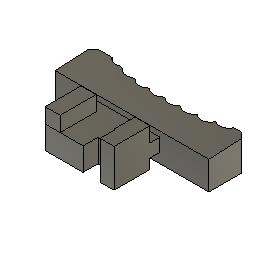
pwrtech_button (Autodesk Fusion 360 design; units mm, degrees)
Autodesk Fusion 360 part; units mm, degrees
note: some values were not read from the file. Chosen so that the rebuilt part matches the saved one: a direction; which face or edge a step refers to; the sign of a taper.
sketch "Sketch1" plane through (0, 0, 0) normal (0, 0, 1) x (1, 0, 0)
  line L0 (0, 0) -> (15.4, 0)
  line L1 (15.4, 0) -> (15.4, -1.3)
  line L2 (0, 0) -> (0, -1.3)
  line L3 (15.4, -1.3) -> (10.5, -1.3)
  line L4 (10.5, -1.3) -> (10.5, -5.9)
  line L5 (0, -1.3) -> (3.6, -1.3)
  line L6 (10.5, -5.9) -> (9, -5.9)
  line L7 (9, -5.9) -> (9, -4.4)
  line L8 (9, -4.4) -> (7.5, -4.4)
  line L9 (7.5, -4.4) -> (7.5, -5.9)
  line L10 (3.6, -1.3) -> (3.6, -5.9)
  line L11 (7.5, -5.9) -> (3.6, -5.9)
  line L12 (10.5, -1.3) -> (10.5, -2.3)
  line L13 (10.5, -2.3) -> (9, -2.3)
  line L14 (9, -2.3) -> (9, -4.4)
  line L15 (9, -4.4) -> (10.5, -4.4)
  line L16 (10.5, -4.4) -> (10.5, -2.3)
  line L17 (3.6, -2.3) -> (5.1, -2.3)
  line L18 (5.1, -2.3) -> (5.1, -4.4)
  line L19 (5.1, -4.4) -> (3.6, -4.4)
  line L20 (3.6, -4.4) -> (3.6, -2.3)
  line L21 (3.6, -1.3) -> (3.6, -3.1)
  line L22 (3.6, -3.1) -> (5.1, -3.1)
  line L23 (5.1, -3.1) -> (5.1, -5.2)
  line L24 (5.1, -5.2) -> (3.6, -5.2)
  line L25 (3.6, -5.2) -> (3.6, -3.1)
  line L26 (10.5, -1.3) -> (10.5, -3.1)
  line L27 (10.5, -3.1) -> (9, -3.1)
  line L28 (9, -3.1) -> (9, -5.2)
  line L29 (9, -5.2) -> (10.5, -5.2)
  line L30 (10.5, -5.2) -> (10.5, -3.1)
  dimension "d1" = 15.4
  dimension "d2" = 1.3
  dimension "d3" = 1.3
  dimension "d4" = 4.9
  dimension "d5" = 4.6
  dimension "d6" = 3.6
  dimension "d7" = 1.5
  dimension "d8" = 1.5
  dimension "d9" = 1.5
  dimension "d10" = 1.5
  dimension "d11" = 1
  dimension "d12" = 1.5
  dimension "d13" = 2.1
  dimension "d14" = 1.8
  dimension "d15" = 1.5
  dimension "d16" = 2.1
  dimension "d17" = 1.8
  dimension "d18" = 1.5
  dimension "d19" = 2.1
  constraint coincident L0.start L2.start
  constraint horizontal L0
  constraint perpendicular L0 L1
  constraint perpendicular L0 L2
  constraint perpendicular L1 L3
  constraint perpendicular L3 L4
  constraint perpendicular L2 L5
  constraint perpendicular L4 L6
  constraint perpendicular L6 L7
  constraint perpendicular L7 L8
  constraint perpendicular L8 L9
  constraint perpendicular L5 L10
  constraint perpendicular L3 L12
  constraint horizontal L13
  constraint vertical L14
  constraint horizontal L15
  constraint vertical L16
  constraint horizontal L17
  constraint vertical L18
  constraint horizontal L19
  constraint vertical L20
  constraint coincident L10 L17.start
  constraint perpendicular L17 L21
  constraint horizontal L22
  constraint vertical L23
  constraint horizontal L24
  constraint vertical L25
  constraint vertical L26
  constraint horizontal L27
  constraint vertical L28
  constraint horizontal L29
  constraint vertical L30
  measures "d1" distance of L0.start L0.end
  measures "d2" distance of L0.end L1.end
  measures "d3" distance of L0.start L2.end
  measures "d4" distance of L1.end L3.end
  measures "d5" distance of L3.end L4.end
  measures "d6" distance of L2.end L5.end
  measures "d7" distance of L4.end L6.end
  measures "d8" distance of L6.end L7.end
  measures "d9" distance of L7.end L8.end
  measures "d10" distance of L8.end L9.end
  measures "d11" distance of L3.end L12.end
  measures "d12" distance of L17.start L17.end
  measures "d13" distance of L17.start L19.end
  measures "d14" distance of L5.end L21.end
  measures "d15" distance of L21.end L22.end
  measures "d16" distance of L21.end L24.end
  measures "d17" distance of L3.end L26.end
  measures "d18" distance of L26.end L27.end
  measures "d19" distance of L26.end L29.end
extrude "Extrude1" add sketch "Sketch1" along normal blind 2 makes body 1
extrude "Extrude2" add sketch "Sketch1" along normal blind 3 contours L10 L17 L18 L20 L21 L22 | L4 L13 L14 L16 L26 L27 | L10 L18 L19 L20 L22 L23 L25 | L4 L14 L15 L16 L27 L28 L30 bodies 1
extrude "Extrude3" cut sketch "Sketch1" along normal blind 0.5 contours L10 L17 L18 L20 L21 L22 | L4 L13 L14 L16 L26 L27 bodies 1
extrude "Extrude4" cut 2 faces at (4.1, -2.3, 0.1667) (10, -2.3, 0.1667) along direction (0, 1, 0) blind 1 on bodies 1 bodies 1
extrude "Extrude5" cut 1 faces at (5.1, -1.9, 0.1667) along direction (1, 0, 0) blind 6.5 on bodies 1 bodies 1
extrude "Extrude6" cut 1 faces at (9, -4.9, 1.3333) along direction (1, 0, 0) blind 0.1 on bodies 1 bodies 1
extrude "Extrude7" cut 1 faces at (7.5, -5.4, 1.3333) along direction (-1, 0, 0) blind 0.1 on bodies 1 bodies 1
extrude "Extrude8" add 1 faces at (5.1333, 0, 0.6667) along direction (0, 1, 0) blind 2.5 on bodies 1 bodies 1
sketch "Sketch2" plane through (0, 0, 2) normal (0, 0, 1) x (-1, 0, 0)
  line L0 (-7.4, 4.4) -> (-9, 4.4)
  line L1 (-9, 4.4) -> (-9, 2.3)
  line L2 (-9, 2.3) -> (-10.5, 2.3)
  line L3 (-10.5, 2.3) -> (-10.5, 1.3)
  line L4 (-10.5, 1.3) -> (-15.4, 1.3)
  line L5 (-15.4, 1.3) -> (-15.4, -2.5)
  line L6 (-15.4, -2.5) -> (0, -2.5)
  line L7 (0, -2.5) -> (0, 1.3)
  line L8 (0, 1.3) -> (-3.6, 1.3)
  line L9 (-3.6, 1.3) -> (-3.6, 2.3)
  line L10 (-3.6, 2.3) -> (-5.1, 2.3)
  line L11 (-5.1, 2.3) -> (-5.1, 4.4)
  line L12 (-5.1, 4.4) -> (-3.6, 4.4)
  line L13 (-3.6, 4.4) -> (-3.6, 5.9)
  line L14 (-3.6, 5.9) -> (-7.4, 5.9)
  line L15 (-7.4, 5.9) -> (-7.4, 4.4)
  spline S0 degree 5 poles (-13.1932, -2.5) (-13.16, -2.4751) (-13.0906, -2.4264) (-12.9777, -2.3563) (-12.8094, -2.2687) (-12.5691, -2.1693) (-12.2987, -2.0801) (-11.9976, -2.0011) (-11.6653, -1.9325) (-11.3014, -1.8744) (-10.9061, -1.8266) (-10.4808, -1.7887) (-10.0277, -1.7597) (-9.551, -1.7384) (-9.0559, -1.723) (-8.5481, -1.712) (-8.0339, -1.7042) (-7.5194, -1.6992) (-7.0101, -1.6972) (-6.5106, -1.6999) (-6.0246, -1.7099) (-5.5551, -1.7299) (-5.1045, -1.7625) (-4.6748, -1.8092) (-4.2679, -1.8704) (-3.8854, -1.9443) (-3.5289, -2.0272) (-3.1998, -2.1149) (-2.8992, -2.2029) (-2.6279, -2.2874) (-2.3864, -2.366) (-2.217, -2.4233) (-2.1033, -2.4629) (-2.0335, -2.4879) (-2, -2.5) knots 0 0 0 0 0 0 0.033333 0.066667 0.1 0.133333 0.166667 0.2 0.233333 0.266667 0.3 0.333333 0.366667 0.4 0.433333 0.466667 0.5 0.533333 0.566667 0.6 0.633333 0.666667 0.7 0.733333 0.766667 0.8 0.833333 0.866667 0.9 0.933333 0.966667 1 1 1 1 1 1
  point P0 (-10.5113, -1.7938)
  point P1 (-4.5685, -1.8279)
  point P2 (-7.415, -1.6993)
  point P3 (-12.319, -2.091)
  point P4 (-2.8487, -2.2195)
  constraint coincident L6 S0.start
  constraint coincident L6 S0.end
extrude "Extrude9" cut sketch "Sketch2" against normal blind 2 contours L6 S0 bodies 1
chamfer "Chamfer1" distance 0.5 angle 45 2 edges at (0, 2.5, 1) (15.4, 2.5, 1) on bodies 1
sketch "Sketch3" plane through (0, 0, 2) normal (0, 0, 1) x (-1, 0, 0)
  line L0 (-15.4, -2) -> (-14.9, -2.5)
  line L1 (-14.9, -2.5) -> (-13.1932, -2.5)
  spline S0 degree 5 poles (-13.1932, -2.5) (-13.16, -2.4751) (-13.0906, -2.4264) (-12.9777, -2.3563) (-12.8094, -2.2687) (-12.5691, -2.1693) (-12.2987, -2.0801) (-11.9976, -2.0011) (-11.6653, -1.9325) (-11.3014, -1.8744) (-10.9061, -1.8266) (-10.4808, -1.7887) (-10.0277, -1.7597) (-9.551, -1.7384) (-9.0559, -1.723) (-8.5481, -1.712) (-8.0339, -1.7042) (-7.5194, -1.6992) (-7.0101, -1.6972) (-6.5106, -1.6999) (-6.0246, -1.7099) (-5.5551, -1.7299) (-5.1045, -1.7625) (-4.6748, -1.8092) (-4.2679, -1.8704) (-3.8854, -1.9443) (-3.5289, -2.0272) (-3.1998, -2.1149) (-2.8992, -2.2029) (-2.6279, -2.2874) (-2.3864, -2.366) (-2.217, -2.4233) (-2.1033, -2.4629) (-2.0335, -2.4879) (-2, -2.5) knots 0 0 0 0 0 0 0.033333 0.066667 0.1 0.133333 0.166667 0.2 0.233333 0.266667 0.3 0.333333 0.366667 0.4 0.433333 0.466667 0.5 0.533333 0.566667 0.6 0.633333 0.666667 0.7 0.733333 0.766667 0.8 0.833333 0.866667 0.9 0.933333 0.966667 1 1 1 1 1 1
  line L2 (-2, -2.5) -> (-0.5, -2.5)
  line L3 (-0.5, -2.5) -> (0, -2)
  line L4 (0, -2) -> (0, 1.3)
  line L5 (0, 1.3) -> (-3.6, 1.3)
  line L6 (-3.6, 1.3) -> (-3.6, 2.3)
  line L7 (-3.6, 2.3) -> (-5.1, 2.3)
  line L8 (-5.1, 2.3) -> (-5.1, 4.4)
  line L9 (-5.1, 4.4) -> (-3.6, 4.4)
  line L10 (-3.6, 4.4) -> (-3.6, 5.9)
  line L11 (-3.6, 5.9) -> (-7.4, 5.9)
  line L12 (-7.4, 5.9) -> (-7.4, 4.4)
  line L13 (-7.4, 4.4) -> (-9, 4.4)
  line L14 (-9, 4.4) -> (-9, 2.3)
  line L15 (-9, 2.3) -> (-10.5, 2.3)
  line L16 (-10.5, 2.3) -> (-10.5, 1.3)
  line L17 (-10.5, 1.3) -> (-15.4, 1.3)
  line L18 (-15.4, 1.3) -> (-15.4, -2)
  line L19 (-10.5, 1.3) -> (-3.6, 1.3)
  constraint coincident L16.end L17.start
  constraint coincident L5.end L6.start
extrude "Extrude10" add sketch "Sketch3" along normal blind 0.6 contours L0 L1 S0 L2 L3 L4 L5 L17 L18 L19 bodies 1
extrude "Extrude11" add 1 faces at (8.2, -3.1, 0.1667) along direction (0, 1, 0) blind 0.6 on bodies 1 bodies 1
extrude "Extrude12" cut 1 faces at (8.2, -2.1, 0.5) along direction (0, 0, 1) blind 0.2 on bodies 1 bodies 1
extrude "Extrude14" add 3 faces at (8.2, -2.7, 0) (4.8667, -4.4667, 0) (7.1854, -0.2971, 0) along direction (0, 0, -1) blind 0.3 on bodies 1 bodies 1
sketch "Sketch6" plane through (0, -4.4, 0) normal (0, -1, 0) x (1, 0, 0)
  line L0 (3.6, 2) -> (5.1, 2)
  line L1 (5.1, 2) -> (5.1, 3)
  line L2 (5.1, 3) -> (3.6, 3)
  line L3 (3.6, 3) -> (3.6, 2)
  line L4 (3.6, 3) -> (5.1, 3)
  line L5 (5.1, 3) -> (5.1, 2)
  line L6 (5.1, 2) -> (3.6, 2)
  line L7 (3.6, 2) -> (3.6, 3)
  line L8 (9, 3) -> (10.5, 3)
  line L9 (10.5, 3) -> (10.5, 2)
  line L10 (10.5, 2) -> (9, 2)
  line L11 (9, 2) -> (9, 3)
  line L12 (9.1, 2) -> (9.1, 3)
  point P0 (9, 3)
  point P1 (10.5, 2)
  point P2 (9.1, 2)
  constraint horizontal L4
  constraint vertical L5
  constraint horizontal L6
  constraint vertical L7
  constraint coincident L0.end L1.start
  constraint coincident L2.end L3.start
  constraint horizontal L8
  constraint vertical L9
  constraint horizontal L10
  constraint vertical L11
  constraint coincident P1 L9.end
  constraint coincident P0 L8.start
  constraint coincident P2 L12.start
  constraint coincident L8 L12.end
  constraint perpendicular L8 L12
extrude "Extrude15" add sketch "Sketch6" along normal blind 1.5 contours L0 L1 L2 L3 L4 L5 L6 L7 | L8 L9 L10 L12 bodies 1
extrude "Extrude16" add 4 faces at (9.5333, -3, 3) (10.0333, -5.4, 3) (4.1, -3, 3) (4.6, -4.9, 3) along direction (0, 0, 1) blind 0.5 on bodies 1 bodies 1
draft "Draft1" angle -3 neutral plane through (0, 0, 0) pull (0, 1, 0) 1 faces at (6.7521, -0.2971, 2.6) on bodies 1
sketch "Sketch5" plane through (0, 0, 0) normal (0, 0, 1) x (1, 0, 0)
  circle A0 centre (-4.7409, 4.224) radius 1
  dimension "d48" = 2
  measures "d48" diameter of A0
extrude "Extrude13" add sketch "Sketch5" along normal blind 3.5 separate body makes body 2
move_body "Move1" bodies 2 to x (1, 0, 0) y (0, 1, 0) z (0, 0, 1) at (6.7409, -1.724, -0.769)
move_body "Move2" bodies 2 to x (1, 0, 0) y (0, 1, 0) z (0, 0, 1) at (0.7, 0.6, 0)
pattern_path "PathPattern1" count 8 spacing 1.5231 from (2.267, 2.4052, 2.7261) backwards along 1 edges at (7.6117, 1.7006, 2.6891) of bodies 2 on bodies 1 makes body 3 at (5.157, 2.5763, 1.5421) makes body 4 at (6.6618, 2.3498, 1.5303) makes body 5 at (8.1835, 2.2938, 1.5273) makes body 6 at (9.7065, 2.3028, 1.5278) makes body 7 at (11.229, 2.3452, 1.53) makes body 8 at (12.7459, 2.4752, 1.5368) makes body 9 at (14.2144, 2.8597, 1.557)
combine "Combine1" operation cut target body 1 tool bodies 2 3 4 9 8 5 6 7
delete_face "DeleteFace1" 1 faces at (13.3959, 2.4062, 2.7236) on bodies 1
delete_face "DeleteFace2" 1 faces at (12.475, 2.0931, 2.7035) on bodies 1
extrude "Extrude17" add 1 faces at (5.9, -2.5, 0.3667) along direction (0, 1, 0) blind 0.2 on bodies 1 bodies 1
equation "d20 = 3 mm - 1 mm"
